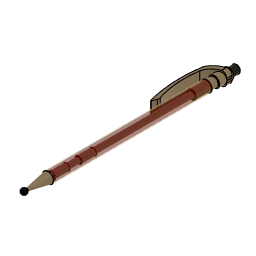
Pen (Autodesk Fusion 360 design; units mm, degrees)
Autodesk Fusion 360 part; units mm, degrees
sketch "Sketch1" plane through (0, 0, 0) normal (0, 1, 0) x (1, 0, 0)
sketch "Sketch2" plane through (0, 0, 0) normal (0, 1, 0) x (1, 0, 0)
  circle A0 centre (0, 0) radius 4.075
  dimension "d5" = 8.15
  constraint coincident A0.centre origin
  measures "d5" diameter of A0
extrude "Extrude1" add sketch "Sketch2" along normal blind 115.75 makes body 1
sketch "Sketch3" plane through (0, 0, 0) normal (0, 1, 0) x (1, 0, 0)
  circle A0 centre (15, 0) radius 2
  dimension "d9" = 4
  measures "d9" diameter of A0
extrude "Extrude2" add sketch "Sketch3" along normal blind 120 separate body makes body 2
sketch "Sketch4" plane through (0, 0, 0) normal (0, -1, 0) x (1, 0, 0)
  circle A0 centre (15, 0) radius 2
ref_plane "WorkPlane1" through (15, 5.15, 0) normal (0, -1, 0) x (1, 0, 0)
sketch "Sketch5" plane through (0, 5.15, 0) normal (0, -1, 0) x (-1, 0, 0)
  circle A0 centre (-15, 0) radius 2
  line L0 (-17.65, -1.53) -> (-15, -3.06)
  line L1 (-15, -3.06) -> (-12.35, -1.53)
  line L2 (-12.35, -1.53) -> (-12.35, 1.53)
  line L3 (-12.35, 1.53) -> (-15, 3.06)
  line L4 (-15, 3.06) -> (-17.65, 1.53)
  line L5 (-17.65, 1.53) -> (-17.65, -1.53)
  point P0 (-15, 0)
  dimension "d13" = 2.65
  constraint coincident P0 A0.centre
  measures "d13" distance of P0 L5
extrude "Extrude3" add sketch "Sketch5" against normal blind 2.5 bodies 2
sketch "Sketch6" plane through (0, 7.65, 0) normal (0, 1, 0) x (-1, 0, 0)
  circle A0 centre (-15, 0) radius 2
  line L0 (-17.65, 1.53) -> (-17.65, -1.53)
  line L1 (-17.65, -1.53) -> (-15, -3.06)
  line L2 (-15, -3.06) -> (-12.35, -1.53)
  line L3 (-12.35, -1.53) -> (-12.35, 1.53)
  line L4 (-12.35, 1.53) -> (-15, 3.06)
  line L5 (-15, 3.06) -> (-17.65, 1.53)
  circle A1 centre (-15, 0) radius 2.5
  dimension "d16" = 5
  constraint concentric A0 A1
  measures "d16" diameter of A1
extrude "Extrude4" add sketch "Sketch6" along normal blind 11 contours A1 bodies 2
ref_plane "WorkPlane2" through (15, 27.4, 0) normal (0, 1, 0) x (-1, 0, 0)
sketch "Sketch7" plane through (0, 27.4, 0) normal (0, 1, 0) x (1, 0, 0)
  circle A0 centre (15, 0) radius 2
  circle A1 centre (15, 0) radius 2.5
  dimension "d20" = 5
  constraint concentric A0 A1
  measures "d20" diameter of A1
extrude "Extrude5" add sketch "Sketch7" along normal blind 10.7 bodies 2
copy_body "Body->Comp1" bodies 2 removing the originals makes body 3 in component "Inside Shaft"
sketch "Sketch1 (2)" plane through (0, 0, 0) normal (0, 1, 0) x (1, 0, 0) in component "Tip"
  circle A0 centre (0, 0) radius 3.875
  dimension "d27" = 7.75
  constraint coincident A0.centre origin
  measures "d27" diameter of A0
ref_plane "WorkPlane1" through (0, -15.5, 0) normal (0, 1, 0) x (1, 0, 0) in component "Tip"
sketch "Sketch2 (2)" plane through (0, -15.5, 0) normal (0, 1, 0) x (1, 0, 0) in component "Tip"
  circle A0 centre (0, 0) radius 1
  dimension "d29" = 2
  constraint coincident A0.centre origin
  measures "d29" diameter of A0
loft "Loft1" add profiles "Sketch1 (2)", "Sketch2 (2)" section 1 section 2 separate body makes body 4 in component "Tip"
extrude "Extrude1'" add 1 faces at (-0.3296, -15.5, -0.5031) along direction (0, -1, 0) blind 2 on bodies 4 bodies 4 in component "Tip"
sketch "Sketch3 (2)" plane through (0, -17.5, 0) normal (0, -1, 0) x (1, 0, 0) in component "Tip"
  circle A0 centre (0, 0) radius 1
  circle A1 centre (0, 0) radius 0.45
  dimension "d32" = 0.9
  constraint coincident A0.centre A1.centre
  measures "d32" diameter of A1
extrude "Extrude2'" cut sketch "Sketch3 (2)" against normal blind 133 contours A1 sketch seen with x (1, 0, 0) y (0, 1, 0) z (0, 0, 1) at (15, 5.15, 0) bodies 3 in component "Inside Shaft"
extrude "Extrude3'" cut sketch "Sketch3 (2)" against normal blind 133 contours A1 bodies 4 in component "Tip"
copy_body "Body->Comp3" bodies 1 removing the originals makes body 5 in component "Housing"
sketch "Sketch1 (3)" plane through (0, 0, 0) normal (0, -1, 0) x (1, 0, 0) in component "Housing"
  circle A0 centre (0, 0) radius 4.075
  circle A1 centre (0, 0) radius 3.65
  dimension "d48" = 7.3
  constraint concentric A0 A1
  measures "d48" diameter of A1
extrude "Extrude1''" cut sketch "Sketch1 (3)" against normal blind 115.75 contours A1 bodies 5 in component "Housing"
sketch "Sketch1 (4)" plane through (0, 120.9, 0) normal (0, 1, 0) x (-1, 0, 0) in component "Clip"
  circle A0 centre (-15, 0) radius 3.65
  circle A1 centre (-15, 0) radius 4.075
  circle A2 centre (-15, 0) radius 3.25
  circle A3 centre (-15, 0) radius 2.35
  dimension "d55" = 6.5
  dimension "d56" = 4.7
  constraint concentric A0 A2
  constraint concentric A2 A3
  measures "d55" diameter of A2
  measures "d56" diameter of A3
extrude "Extrude1'''" add sketch "Sketch1 (4)" along normal blind 16.45 separate body contours A2 makes body 6 in component "Clip"
sketch "Sketch2 (3)" plane through (0, 137.35, 0) normal (0, 1, 0) x (-1, 0, 0) in component "Clip"
  circle A0 centre (-15, 0) radius 2.35
  circle A1 centre (-15, 0) radius 3.25
  circle A2 centre (-15, 0) radius 4
  dimension "d59" = 8
  constraint concentric A0 A2
  measures "d59" diameter of A2
extrude "Extrude2''" add sketch "Sketch2 (3)" along normal blind 10.3 separate body contours A2 makes body 7 in component "Clip"
ref_plane "WorkPlane1" through (15, 142.5, 0) normal (0, 0, 1) x (0, 1, 0) in component "Clip"
sketch "Sketch3 (3)" plane through (0, 0, 0) normal (0, 0, 1) x (1, 0, 0) in component "Clip"
sketch "Sketch4 (2)" plane through (0, 0, 0) normal (0, 0, 1) x (1, 0, 0) in component "Clip"
  arc A0 (19.0438, 146.4176) -> (6.6949, 138.3567) centre (20.2574, 131.0691) ccw
  arc A1 (6.6949, 138.3567) -> (8.8968, 96.5196) centre (101.007, 122.3438) ccw
  line L0 (8.8968, 96.5196) -> (10.7717, 101.5267)
  arc A2 (7.9315, 133.863) -> (10.7717, 101.5267) centre (75.5436, 123.5087) ccw
  arc A3 (18.9981, 142.5001) -> (7.9315, 133.863) centre (18.579, 131.6288) ccw
  line L1 (18.9981, 142.5001) -> (18.9981, 146.4139)
  line L2 (18.9981, 146.4139) -> (19.0438, 146.4176)
  constraint vertical L1
  constraint coincident A0 L1.end
extrude "Extrude3''" add sketch "Sketch4 (2)" along normal mid plane 10 separate body makes body 8 in component "Clip"
fillet "Fillet1" radius 3.5 1 edges at (18.9981, 144.457, 5) on bodies 8 in component "Clip"
fillet "Fillet1" radius 3.5 1 edges at (18.9981, 144.457, -5) on bodies 8 in component "Clip"
fillet "Fillet2" radius 0.25 1 edges at (8.8968, 96.5196, 0) on bodies 8 in component "Clip"
fillet "Fillet3" radius 3.125 1 edges at (10.7717, 101.5267, 0) on bodies 8 in component "Clip"
combine "Combine1" operation add target body 6 tool bodies 7 8 in component "Clip"
sketch "Sketch8" plane through (0, 126.45, 0) normal (0, 1, 0) x (-1, 0, 0)
  circle A0 centre (-15, 0) radius 2.35
  circle A1 centre (-15, 0) radius 3.25
  circle A2 centre (-15, 0) radius 3.25
  constraint concentric A0 A2
sketch "Sketch9" plane through (0, 136.75, 0) normal (0, 1, 0) x (-1, 0, 0)
  circle A0 centre (-15, 0) radius 3.25
  circle A1 centre (-15, 0) radius 4
  circle A2 centre (-15, 0) radius 3.25
  constraint concentric A0 A2
extrude "Extrude4'" cut sketch "Sketch9" against normal blind 10.35 contours A0 A2 sketch seen with x (1, 0, 0) y (0, 1, 0) z (0, 0, 1) at (0, 10.9, 0) bodies 6 makes body 9 at (11.7662, 131.8333, -0.3236) in component "Clip"
sketch "Sketch1 (5)" plane through (0, 147.65, 0) normal (0, 1, 0) x (-1, 0, 0) in component "Eraser"
  circle A0 centre (-15, 0) radius 3.25
  circle A1 centre (-15, 0) radius 4
  circle A2 centre (-15, 0) radius 3.1
  dimension "d82" = 6.2
  constraint concentric A0 A2
  measures "d82" diameter of A2
extrude "Extrude1''''" add sketch "Sketch1 (5)" along normal blind -10.5 and the other way blind -7 separate body contours A2 makes body 10 in component "Eraser"
fillet "Fillet1'" radius 1.5 1 edges at (17.8902, 154.65, -1.121) on bodies 10 in component "Eraser"
component "Tip" placed x (1, 0, 0) y (0, 1, 0) z (0, 0, 1) at (15, 5.15, 0)
component "Inside Shaft" placed x (1, 0, 0) y (0, 1, 0) z (0, 0, 1) at (0, 0, 0)
component "Housing" placed x (1, 0, 0) y (0, 1, 0) z (0, 0, 1) at (15, 5.15, 0)
component "Clip" placed x (1, 0, 0) y (0, 1, 0) z (0, 0, 1) at (0, -10.9, 0)
component "Eraser" placed x (1, 0, 0) y (0, 1, 0) z (0, 0, 1) at (0, 0, 0) in component "Clip"
